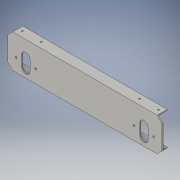
# Autodesk Inventor part: ChassisSideBracket
Saved by Autodesk Inventor 2016 (Build 200138000, 138)
## iProperties
Created: 2015-08-06
Part Number: ChassisSideBracket
Material: Generic
Document SubType Name: Modeling
Designer: lachesis
Density: 1 g/cm^3
Appearance: Default
Author: lachesis
Autodesk Inventor part; units mm, degrees
ref_plane "YZ Plane" through (0, 0, 0) normal (1, 0, 0) x (0, 1, 0)
ref_plane "XZ Plane" through (0, 0, 0) normal (0, 1, 0) x (-1, 0, 0)
ref_plane "XY Plane" through (0, 0, 0) normal (0, 0, 1) x (1, 0, 0)
sketch "Sketch1" plane through (0, 0, 0) normal (0, 0, 1) x (1, 0, 0)
  line L0 (-114.2436, 26.55) -> (114.2436, 26.55)
  line L1 (122, 18.7501) -> (122, -18.7501)
  line L2 (114.2436, -26.55) -> (-114.2436, -26.55)
  line L3 (-122, -18.7501) -> (-122, 18.7501)
  line L4 (114.2436, 26.55) -> (122, 18.7501)
  line L5 (122, -18.7501) -> (114.2436, -26.55)
  line L6 (0, 26.55) -> (0, -26.55)
  line L7 (-114.2436, 26.55) -> (-122, 18.7501)
  line L8 (-122, -18.7501) -> (-114.2436, -26.55)
  point P0 (0, 0)
  point P1 (-122, 0)
  point P2 (0, 26.55)
  point P3 (0, 0)
  dimension "d0" = 244
  dimension "d62" = 135.16
  dimension "d63" = 11
  dimension "d64" = 135.16
  dimension "d65" = 11
  dimension "d66" = 53.1
  constraints: 18 end point, 5 midpoint, 4 symmetric about line, 2 parallel, 1 coincident, 1 horizontal, 1 horizontal alignment, 1 perpendicular, 1 vertical alignment
  measures "d0" distance of L3.end L1.start
  measures "d62" angle of L1 L4
  measures "d63" distance of L0.end L1.start
  measures "d64" angle of L1 L5
  measures "d65" distance of L2.start L1.end
  measures "d66" distance between parallel lines of L2 L0
extrude "Extrusion5" add sketch "Sketch1" along normal blind 1.6
sketch "Sketch11" plane through (-114.2436, 26.55, 0) normal (0, 1, 0) x (1, 0, 0)
  line L0 (228.4872, 0) -> (0, 0) projected
  line L1 (0, 0) -> (0, -1.6) projected
  line L2 (228.4872, -1.6) -> (0, -1.6) projected
  line L3 (228.4872, 0) -> (228.4872, -1.6) projected
  line L4 (228.4872, 0) -> (0, 0) projected
  line L5 (0, 0) -> (228.4872, 0)
  line L6 (228.4872, 0) -> (228.4872, 14.4)
  line L7 (228.4872, 14.4) -> (0, 14.4)
  line L8 (0, 14.4) -> (0, 0)
  point P0 (114.2436, 0)
  dimension "d72" = 14.4
  constraints: 8 end point, 2 parallel, 1 horizontal, 1 perpendicular
  measures "d72" distance of L0.start L6.end
extrude "Extrusion6" add sketch "Sketch11" against normal blind 1.6 contours L0 L8 L7 L6
sketch "Sketch12" plane through (-114.2436, -26.55, 0) normal (0, -1, 0) x (1, 0, 0)
  line L0 (228.4872, -14.4) -> (228.4872, 0) projected
  line L1 (0, 0) -> (228.4872, 0) projected
  line L2 (0, 0) -> (0, -14.4) projected
  line L3 (0, -14.4) -> (228.4872, -14.4) projected
  line L4 (0, 0) -> (228.4872, 0) projected
  line L5 (0, 0) -> (228.4872, 0)
  line L6 (228.4872, 0) -> (228.4872, -14.4)
  line L7 (228.4872, -14.4) -> (0, -14.4)
  line L8 (0, -14.4) -> (0, 0)
  point P0 (114.2436, 0)
  constraints: 8 end point, 2 parallel, 1 horizontal, 1 perpendicular
extrude "Extrusion7" add sketch "Sketch12" against normal blind 1.6
sketch "Sketch13" plane through (-114.2436, 26.55, 1.6) normal (0, 1, 0) x (1, 0, 0)
  line L0 (0, 1.6) -> (0, 0) projected
  line L1 (228.4872, 0) -> (0, 0) projected
  line L2 (228.4872, 1.6) -> (228.4872, 0) projected
  line L3 (228.4872, 1.6) -> (228.4872, 16) projected
  line L4 (228.4872, 16) -> (0, 16) projected
  line L5 (0, 16) -> (0, 1.6) projected
  point P0 (114.2436, 1.6)
  point P1 (36.4, 8.8)
  point P2 (192.0872, 8.8)
  point P3 (0, 8.8)
  point P4 (6.354, 8.8)
  point P5 (222.1332, 8.8)
  dimension "d77" = 36.4
  dimension "d78" = 36.4
  dimension "d79" = 6.354
  dimension "d80" = 6.354
  constraints: 5 horizontal alignment, 1 midpoint
  measures "d77" distance from line of L5 point (36.4, 8.8)
  measures "d78" distance from line of L3 point (192.087, 8.8)
  measures "d79" distance from line of L5 point (6.354, 8.8)
  measures "d80" distance from line of L3 point (222.133, 8.8)
hole "Hole6" at (-77.8436, 26.55, -7.2) at (77.8436, 26.55, -7.2) at (-107.8896, 26.55, -7.2) at (107.8896, 26.55, -7.2) direction (0, -1, 0) diameter 2.459 end up to face face through (38.0812, 24.95, -4.8) facing (0, -1, 0) thread size "M3x0.5" class "6H" standard "ISO Metric profile"
sketch "Sketch14" plane through (-114.2436, -26.55, 1.6) normal (0, -1, 0) x (1, 0, 0)
  circle A0 centre (192.0872, -8.8) radius 1.2295 projected
  circle A1 centre (222.1332, -8.8) radius 1.2295 projected
  circle A2 centre (36.4, -8.8) radius 1.2295 projected
  circle A3 centre (6.354, -8.8) radius 1.2295 projected
  point P0 (114.2436, -1.6)
  constraints: 4 coincident
hole "Hole7" at (-107.8896, -26.55, -7.2) at (-77.8436, -26.55, -7.2) at (77.8436, -26.55, -7.2) at (107.8896, -26.55, -7.2) direction (0, 1, 0) diameter 2.459 end up to face face through (38.0812, -24.95, -9.6) facing (0, 1, 0) thread size "M3x0.5" class "6H" standard "ISO Metric profile"
sketch "Sketch15" plane through (0, 0, 1.6) normal (0, 0, 1) x (1, 0, 0)
  line L0 (-93.5, 2.55) -> (-93.5, -14.45) construction
  line L1 (-100, 2.55) -> (-100, -14.45)
  line L2 (-87, -14.45) -> (-87, 2.55)
  arc A0 (-87, 2.55) -> (-100, 2.55) centre (-93.5, 2.55) ccw
  arc A1 (-100, -14.45) -> (-87, -14.45) centre (-93.5, -14.45) ccw
  line L3 (-122, 18.7501) -> (-122, -18.7501) projected
  line L4 (114.2436, 26.55) -> (-114.2436, 26.55) projected
  line L5 (0, 26.55) -> (0, -26.55)
  line L6 (-114.2436, -26.55) -> (114.2436, -26.55) projected
  line L7 (93.5, 2.55) -> (93.5, -14.45) construction
  line L8 (100, 2.55) -> (100, -14.45)
  line L9 (87, -14.45) -> (87, 2.55)
  arc A2 (100, 2.55) -> (87, 2.55) centre (93.5, 2.55) ccw
  arc A3 (87, -14.45) -> (100, -14.45) centre (93.5, -14.45) ccw
  point P0 (0, 0)
  point P1 (-93.5, -5.95)
  point P2 (93.5, -5.95)
  dimension "d95" = 17
  dimension "d96" = 13
  dimension "d97" = 22
  dimension "d98" = 24
  constraints: 18 end point, 8 point on circle, 7 symmetric about line, 4 centre point, 4 tangent, 3 midpoint, 1 parallel, 1 vertical, 2 other
  measures "d95" distance of L0.start L0.end
  measures "d96" diameter of A1
  measures "d97" distance between parallel lines of L3 L1
  measures "d98" distance from line of L4 L0.start
extrude "Extrusion8" cut sketch "Sketch15" against normal through all
sketch "Sketch16" plane through (0, 0, 1.6) normal (0, 0, 1) x (1, 0, 0)
  line L0 (-109, -5.95) -> (-78, -5.95)
  line L1 (78, -5.95) -> (109, -5.95)
  arc A0 (-87, 2.55) -> (-100, 2.55) centre (-93.5, 2.55) ccw projected
  arc A1 (100, 2.55) -> (87, 2.55) centre (93.5, 2.55) ccw projected
  line L2 (-87, 2.55) -> (-87, -14.45) projected
  point P0 (0, 0)
  point P1 (-93.5, -5.95)
  point P2 (93.5, -5.95)
  point P3 (-87, -5.95)
  dimension "d101" = 31
  dimension "d102" = 31
  constraints: 4 end point, 3 midpoint, 2 horizontal, 2 horizontal alignment, 2 vertical alignment
  measures "d101" distance of L0.end L0.start
  measures "d102" distance of L1.end L1.start
hole "Hole8" at (-109, -5.95, 1.6) at (-78, -5.95, 1.6) at (78, -5.95, 1.6) at (109, -5.95, 1.6) direction (0, 0, -1) diameter 3 end through all
equation "\"d64\" = d62"
equation "\"d78\" = d77"
equation "\"d79\" = d80"
body "Solid1"
body "Solid2"
